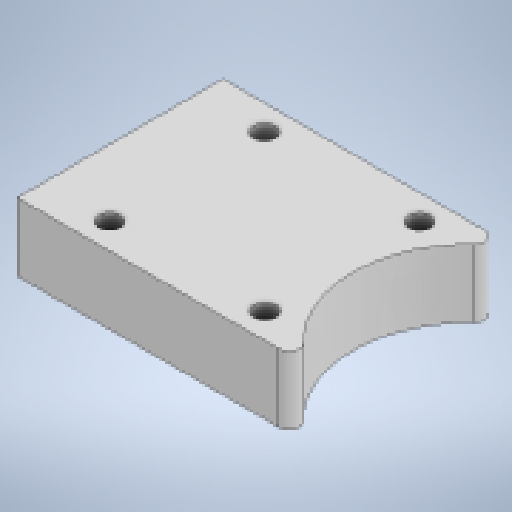
# Autodesk Inventor part: 3D_printed_part
Saved by Autodesk Inventor 2025.2 (Build 292293000, 293)
## iProperties
Created: 2025-05-14
Part Number: 3D_printed_part
Material: Generic
Document SubType Name: Modeling
Designer: User
Density: 1 g/cm^3
Appearance: Default
Author: User
Autodesk Inventor part; units mm, degrees
ref_plane "YZ Plane" through (0, 0, 0) normal (1, 0, 0) x (0, 1, 0)
ref_plane "XZ Plane" through (0, 0, 0) normal (0, 1, 0) x (-1, 0, 0)
ref_plane "XY Plane" through (0, 0, 0) normal (0, 0, 1) x (1, 0, 0)
sketch "Sketch1" plane through (0, 0, 0) normal (0, 1, 0) x (-1, 0, 0)
  line L0 (4, 10) -> (-19.4211, 10)
  line L1 (-19.4211, -10) -> (4, -10)
  line L2 (4, -10) -> (4, 10)
  arc A0 (-19.4211, -10) -> (-19.4211, 10) centre (-25.1, 0) ccw
  line L3 (4, -10) -> (9, -10)
  line L4 (9, -10) -> (9, 10)
  line L5 (9, 10) -> (4, 10)
  line L6 (4, 10) -> (4, -10)
  point P0 (0, 0)
  dimension "d0" = 20
  dimension "d2" = 4
  dimension "d3" = 10
  dimension "d6" = 10
  dimension "d7" = 23
  dimension "d8" = 29.1
  dimension "d11" = 23.4211
  dimension "d12" = 20
  dimension "d13" = 5
  constraints: 14 end point, 3 parallel, 2 horizontal, 2 point on circle, 1 centre point, 1 perpendicular
  measures "d0" distance of L1.end L0.start
  measures "d2" distance from line of point (0, 0) L2
  measures "d3" distance from line of point (0, 0) L0
  measures "d6" distance from line of L1 A0.centre
  measures "d7" diameter of A0
  measures "d8" distance from line of L2 A0.centre
  measures "d11" distance of L1.start L1.end
  measures "d12" distance of L3.end L4.end
  measures "d13" distance of L4.end L5.end
extrude "Extrusion1" add sketch "Sketch1" along normal blind 6.61
fillet "Fillet1" radius 1 2 edges at (19.4211, 3.305, -10) (19.4211, 3.305, 10)
sketch "Sketch2" plane through (0, 0, 0) normal (0, -1, 0) x (1, 0, 0)
  circle A0 centre (-2.5, 7.525) radius 0.7835 projected
  circle A1 centre (-2.5, -7.525) radius 0.7835 projected
  circle A2 centre (12.6, -7.525) radius 0.7835 projected
  circle A3 centre (12.6, 7.525) radius 0.7835 projected
  point P0 (0, 0)
hole "Hole1" at (-2.5, 0, -7.525) at (-2.5, 0, 7.525) at (12.6, 0, 7.525) at (12.6, 0, -7.525) direction (0, 1, 0) diameter 2.1 depth 6.61
body "Solid1"
